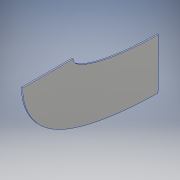
# Autodesk Inventor part: Storage Side Plate
Saved by Autodesk Inventor 2019.4 (Build 234330000, 330)
## iProperties
Created: 2020-01-11
Part Number: Storage Side Plate
Material: Aluminum 6061
Document SubType Name: Modeling
Designer: admin
Density: 2.7 g/cm^3
Appearance: Aluminum - Flat
Author: admin
Autodesk Inventor part; units mm, degrees
ref_plane "YZ Plane" through (0, 0, 0) normal (1, 0, 0) x (0, 1, 0)
ref_plane "XZ Plane" through (0, 0, 0) normal (0, 1, 0) x (-1, 0, 0)
ref_plane "XY Plane" through (0, 0, 0) normal (0, 0, 1) x (1, 0, 0)
sketch "Sketch1" plane through (0, 0, 0) normal (1, 0, 0) x (0, 1, 0)
  line L0 (0, 0) -> (-46.627, 0) construction
  line L1 (-46.627, 0) -> (-85.022, -162.7653) construction
  line L2 (-85.022, -162.7653) -> (-87.1277, -345.1668) construction
  spline S0 degree 3 poles (0, 0) (-46.627, 0) (-85.022, -162.7653) (-87.1277, -345.1668) knots 1 1 1 1 2 2 2 2
  line L3 (0, 203.2) -> (0, 0)
  line L4 (-290.3141, -342.8213) -> (-87.1277, -345.1668)
  spline S1 degree 5 poles (0, 203.2) (-30.0832, 203.1994) (-60.163, 198.1349) (-89.1135, 187.9906) (-132.1139, 164.2585) (-167.6593, 130.8983) (-179.9619, 117.021) (-198.9007, 91.6349) (-214.4712, 64.1013) (-220.3955, 52.3535) (-230.6822, 29.6716) (-239.3899, 6.3414) (-243.1882, -4.7821) (-250.2288, -27.1972) (-256.2764, -49.9002) (-259.0793, -61.3034) (-264.3893, -84.6463) (-268.9425, -108.1487) (-271.0846, -120.1568) (-275.1318, -144.795) (-278.5301, -169.5312) (-280.1101, -182.2045) (-283.0304, -208.1305) (-285.3472, -234.1176) (-286.3791, -247.3967) (-288.1801, -274.4329) (-289.3843, -301.5023) (-289.845, -315.272) (-290.1551, -329.0458) (-290.3141, -342.8213) knots 0 0 0 0 0 0 0.219224 0.219224 0.219224 0.353657 0.353657 0.353657 0.449419 0.449419 0.449419 0.535041 0.535041 0.535041 0.620599 0.620599 0.620599 0.70948 0.70948 0.70948 0.802545 0.802545 0.802545 0.899602 0.899602 0.899602 1 1 1 1 1 1
  dimension "d0" = 203.2
  constraints: 4 end point, 1 vertical, 6 other
extrude "Extrusion1" add sketch "Sketch1" along normal blind 5
body "Solid1"
